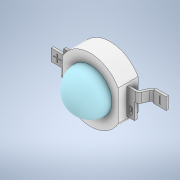
# Autodesk Inventor part: Part1
Saved by Autodesk Inventor 2022 (Build 260153000, 153)
## iProperties
Created: 2023-08-05
Part Number: Part1
Material: Generic
Document SubType Name: Modeling
Designer: danil
Density: 1 g/cm^3
Appearance: Default
Author: danil
Autodesk Inventor part; units mm, degrees
ref_plane "YZ Plane" through (0, 0, 0) normal (1, 0, 0) x (0, 1, 0)
ref_plane "XZ Plane" through (0, 0, 0) normal (0, 1, 0) x (-1, 0, 0)
ref_plane "XY Plane" through (0, 0, 0) normal (0, 0, 1) x (1, 0, 0)
sketch "Sketch1" plane through (0, 0, 0) normal (0, 0, 1) x (1, 0, 0)
  circle A0 centre (0, 0) radius 2.9
  dimension "d0" = 5.8
  constraints: 1 centre point, 1 coincident
  measures "d0" diameter of A0
extrude "Extrusion1" add sketch "Sketch1" along normal blind 0.1
sketch "Sketch2" plane through (0, 0, 0.1) normal (0, 0, 1) x (1, 0, 0)
  circle A0 centre (0, 0) radius 4
  line L0 (-3.5, 1.9365) -> (3.5, 1.9365)
  line L1 (3.5, 1.9365) -> (3.5, -1.9365)
  line L2 (3.5, -1.9365) -> (-3.5, -1.9365)
  line L3 (-3.5, -1.9365) -> (-3.5, 1.9365)
  point P0 (-3.5, -1.9365)
  dimension "d3" = 8
  dimension "d4" = 7
  constraints: 8 end point, 3 point on circle, 2 parallel, 1 centre point, 1 coincident, 1 horizontal, 1 perpendicular
  measures "d3" diameter of A0
  measures "d4" distance between parallel lines of L1 L3
extrude "Extrusion2" add sketch "Sketch2" along normal blind 2.5 separate body contours L0 A0 | L1 L2 L3 L0 | A0 L2
fillet "Fillet1" radius 0.1 1 edges at (-2.9, 0, 0)
sketch "Sketch3" plane through (0, 0, 2.6) normal (0, 0, 1) x (1, 0, 0)
  circle A0 centre (0, 0) radius 2.7
  dimension "d8" = 5.4
  constraints: 1 centre point, 1 coincident
  measures "d8" diameter of A0
extrude "Extrusion3" add sketch "Sketch3" along normal blind 2.7 separate body
fillet "Fillet2" radius 2.7 1 edges at (-2.7, 0, 5.3)
sketch "Sketch4" plane through (0, 0, 0) normal (0, 1, 0) x (-1, 0, 0)
  line L0 (7.25, 0) -> (5.25, 0)
  line L1 (5.25, 0) -> (4.7065, 1.2)
  line L2 (4.7065, 1.2) -> (3.5, 1.2)
  line L3 (7.25, 0.3) -> (5.4435, 0.3)
  line L4 (5.4435, 0.3) -> (4.9, 1.5)
  line L5 (4.9, 1.5) -> (3.5, 1.5)
  line L6 (7.25, 0.3) -> (7.25, 0)
  line L7 (3.5, 1.5) -> (3.5, 1.2)
  line L8 (0, 0) -> (0, 5.7322) construction
  line L9 (-7.25, 0) -> (-5.25, 0)
  line L10 (-5.25, 0) -> (-4.7065, 1.2)
  line L11 (-4.7065, 1.2) -> (-3.5, 1.2)
  line L12 (-7.25, 0.3) -> (-5.4435, 0.3)
  line L13 (-5.4435, 0.3) -> (-4.9, 1.5)
  line L14 (-4.9, 1.5) -> (-3.5, 1.5)
  line L15 (-7.25, 0.3) -> (-7.25, 0)
  line L16 (-3.5, 1.5) -> (-3.5, 1.2)
  dimension "d12" = 0.3
  dimension "d14" = 0.3
  dimension "d16" = 0.3
  dimension "d17" = 3.5
  dimension "d18" = 1.5
  dimension "d20" = 2
  dimension "d21" = 1.4
  dimension "d29" = 14.5
  constraints: 34 end point, 8 symmetric about line, 2 horizontal, 2 parallel, 2 perpendicular, 1 point on line, 1 vertical
  measures "d12" distance between parallel lines of L2 L5
  measures "d14" distance between parallel lines of L0 L3
  measures "d16" distance between parallel lines of L1 L4
  measures "d17" distance from line of L8.start L7
  measures "d18" distance from line of L8.start L5
  measures "d20" distance from line of L0.end L6
  measures "d21" distance from line of L4.end L7
  measures "d29" distance between parallel lines of L6 L15
extrude "Extrusion4" add sketch "Sketch4" along normal mid plane 3.4 separate body
fillet "Fillet3" radius 0.3 4 edges at (-4.7065, 0, 1.2) (-5.4435, 0, 0.3) (4.7065, 0, 1.2) (5.4435, 0, 0.3)
fillet "Fillet4" radius 0.5 4 edges at (-4.9, 0, 1.5) (-5.25, 0, 0) (4.9, 0, 1.5) (5.25, 0, 0)
sketch "Sketch5" plane through (-7.25, -1.7, 0) normal (0, 0, -1) x (-1, 0, 0)
  line L0 (-2.75, 3.4) -> (-2.75, 1.35)
  line L1 (-2.75, 1.35) -> (-1.7, 1.35)
  line L2 (-1.7, 1.35) -> (-1.55, 1.5)
  line L3 (-1.55, 1.5) -> (0, 1.5)
  line L4 (0, 1.5) -> (0, 0)
  line L5 (0, 0) -> (-1.55, 0)
  line L6 (-1.55, 0) -> (-1.7, 0.15)
  line L7 (-1.7, 0.15) -> (-3.75, 0.15)
  line L8 (-1.7, 1.35) -> (-1.7, 0.15) construction
  line L9 (-2.75, 3.4) -> (-3.75, 3.4)
  line L10 (-14.5, 3.4) -> (-12.95, 3.4)
  line L11 (-12.95, 3.4) -> (-12.8, 3.25)
  line L12 (-12.8, 3.25) -> (-10.75, 3.25)
  line L13 (-10.75, 0) -> (-11.75, 0)
  line L14 (-11.75, 0) -> (-11.75, 2.05)
  line L15 (-11.75, 2.05) -> (-12.8, 2.05)
  line L16 (-12.8, 2.05) -> (-12.95, 1.9)
  line L17 (-12.95, 1.9) -> (-14.5, 1.9)
  line L18 (-14.5, 1.9) -> (-14.5, 3.4)
  line L19 (-3.75, 3.4) -> (-3.75, 0.15)
  line L20 (-10.75, 3.25) -> (-10.75, 0)
  line L21 (0, 0) -> (-14.5, 0)
  line L22 (-14.5, 0) -> (-14.5, 3.4)
  line L23 (-14.5, 3.4) -> (0, 3.4)
  line L24 (0, 3.4) -> (0, 0)
  line L25 (-11.25, 1.2) -> (-11.25, 0.6) construction
  line L26 (-11.05, 1.2) -> (-11.05, 0.6)
  line L27 (-11.45, 0.6) -> (-11.45, 1.2)
  arc A0 (-11.05, 1.2) -> (-11.45, 1.2) centre (-11.25, 1.2) ccw
  arc A1 (-11.45, 0.6) -> (-11.05, 0.6) centre (-11.25, 0.6) ccw
  point P0 (-1.7, 0.75)
  point P1 (0, 0.75)
  point P2 (-11.25, 0.9)
  point P3 (-11.25, 0)
  point P4 (-3.75, 3.4)
  point P5 (-10.75, 0)
  point P6 (0, 1.5)
  point P7 (-2.75, 3.4)
  point P8 (-11.75, 0)
  dimension "d31" = 1.5
  dimension "d32" = 1.2
  dimension "d33" = 135
  dimension "d34" = 1.7
  dimension "d35" = 1
  dimension "d36" = 3.4
  dimension "d37" = 3.75
  dimension "d38" = 7
  dimension "d39" = 1
  dimension "d41" = 0.4
  dimension "d42" = 0.6
  constraints: 58 end point, 16 parallel, 10 perpendicular, 4 midpoint, 4 point on circle, 4 tangent, 3 vertical, 2 centre point, 2 horizontal, 2 vertical alignment, 1 collinear, 1 horizontal alignment, 1 other
  measures "d31" distance between parallel lines of L5 L3
  measures "d32" distance between parallel lines of L7 L1
  measures "d33" angle of L3 L2
  measures "d34" horizontal distance of L1.end point (0, 0.75)
  measures "d35" distance between parallel lines of L19 L0
  measures "d36" distance between parallel lines of L5 L9
  measures "d37" distance between parallel lines of L19 L4
  measures "d38" distance between parallel lines of L20 L19
  measures "d41" distance between parallel lines of L27 L26
  measures "d42" distance of point (-11.25, 0) L25.end
extrude "Extrusion5" cut sketch "Sketch5" against normal through all contours L23 L24 L3 L2 L1 L0 | L19 L7 L6 L21 L20 L12 L11 L23 | L17 L16 L15 L14 L21 L22 | L26 A1 L27 A0 bodies 4
sketch "Sketch6" plane through (-7.25, -0.2, 0.3) normal (0, 0, 1) x (1, 0, 0)
  line L0 (0.775, -0.3) -> (0.775, -1.2) construction
  line L1 (0.725, -0.3) -> (0.725, -1.2)
  line L2 (0.825, -1.2) -> (0.825, -0.3)
  arc A0 (0.825, -0.3) -> (0.725, -0.3) centre (0.775, -0.3) ccw
  arc A1 (0.725, -1.2) -> (0.825, -1.2) centre (0.775, -1.2) ccw
  line L3 (0, -1.5) -> (0, 0) projected
  line L4 (0.325, -0.75) -> (1.225, -0.75) construction
  line L5 (0.325, -0.8) -> (1.225, -0.8)
  line L6 (1.225, -0.7) -> (0.325, -0.7)
  arc A2 (0.325, -0.7) -> (0.325, -0.8) centre (0.325, -0.75) ccw
  arc A3 (1.225, -0.8) -> (1.225, -0.7) centre (1.225, -0.75) ccw
  line L7 (1.55, 0) -> (0, 0) projected
  line L8 (13.725, 1.6) -> (13.725, 0.7) construction
  line L9 (13.675, 1.6) -> (13.675, 0.7)
  line L10 (13.775, 0.7) -> (13.775, 1.6)
  arc A4 (13.775, 1.6) -> (13.675, 1.6) centre (13.725, 1.6) ccw
  arc A5 (13.675, 0.7) -> (13.775, 0.7) centre (13.725, 0.7) ccw
  line L11 (14.5, 0.4) -> (14.5, 1.9) projected
  line L12 (12.95, 1.9) -> (14.5, 1.9) projected
  point P0 (7.25, 0.2)
  point P1 (0.775, -0.75)
  point P2 (0, -0.75)
  point P3 (0.775, -0.75)
  point P4 (0.775, 0)
  point P5 (13.725, 1.15)
  point P6 (14.5, 1.15)
  point P7 (13.725, 1.9)
  point P8 (0.825, -0.7)
  point P9 (0.725, -0.7)
  point P10 (0.725, -0.8)
  point P11 (0.825, -0.8)
  dimension "d45" = 0.1
  dimension "d46" = 1
  dimension "d47" = 0.1
  dimension "d48" = 1
  dimension "d49" = 0.1
  dimension "d50" = 1
  constraints: 24 end point, 12 point on circle, 12 tangent, 7 midpoint, 6 centre point, 3 parallel, 2 horizontal alignment, 2 vertical, 2 vertical alignment, 1 coincident, 1 perpendicular
  measures "d45" diameter of A1
  measures "d47" diameter of A3
  measures "d49" diameter of A5
extrude "Extrusion6" cut sketch "Sketch6" against normal blind 0.01 bodies 4
chamfer "Chamfer1" distance 0.05 angle 45 2 edges at (-4.5, 1.7, 1.35) (4.5, -1.7, 1.35)
equation "\"d14\" = d12"
equation "\"d16\" = d12"
equation "\"d47\" = d45"
equation "\"d48\" = d46"
equation "\"d49\" = d45"
equation "\"d50\" = d46"
